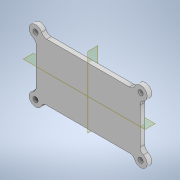
# Autodesk Inventor part: sensor_lid
Saved by Autodesk Inventor 2020 (Build 240168000, 168)
## iProperties
Created: 2020-03-10
Part Number: sensor_lid
Material: Generic
Document SubType Name: Modeling
Designer: Richard
Density: 1 g/cm^3
Appearance: Default
Author: Richard
Autodesk Inventor part; units mm, degrees
ref_plane "YZ Plane" through (0, 0, 0) normal (1, 0, 0) x (0, 1, 0)
ref_plane "XZ Plane" through (0, 0, 0) normal (0, 1, 0) x (-1, 0, 0)
ref_plane "XY Plane" through (0, 0, 0) normal (0, 0, 1) x (1, 0, 0)
sketch "Sketch1" plane through (0, 0, 0) normal (0, 0, 1) x (1, 0, 0)
  line L0 (-172.0273, 68.4234) -> (-119.9573, 68.4234)
  line L1 (-119.9573, 68.4234) -> (-119.9573, 42.0074)
  line L2 (-119.9573, 42.0074) -> (-172.0273, 42.0074)
  line L3 (-172.0273, 42.0074) -> (-172.0273, 68.4234)
  point P0 (0, 0)
  dimension "d0" = 52.07
  dimension "d1" = 26.416
  constraints: 8 end point, 2 parallel, 1 horizontal, 1 perpendicular
  measures "d0" distance of L1.end L2.end
  measures "d1" distance of L0.end L1.end
extrude "Extrusion1" add sketch "Sketch1" along normal blind 2.54
sketch "Sketch2" plane through (0, 0, 2.54) normal (0, 0, 1) x (1, 0, 0)
  line L0 (-119.9573, 68.4234) -> (-172.0273, 68.4234) projected
  line L1 (-119.9573, 68.4234) -> (-172.0273, 68.4234) projected
  line L2 (-172.0273, 68.4234) -> (-172.0273, 42.0074) projected
  line L3 (-172.0273, 42.0074) -> (-119.9573, 42.0074) projected
  line L4 (-119.9573, 42.0074) -> (-119.9573, 68.4234) projected
  line L5 (-174.5673, 39.4674) -> (-174.5673, 70.9634)
  line L6 (-174.5673, 70.9634) -> (-117.4173, 70.9634)
  line L7 (-117.4173, 70.9634) -> (-117.4173, 39.4674)
  line L8 (-117.4173, 39.4674) -> (-174.5673, 39.4674)
  point P0 (0, 0)
  dimension "d4" = 2.54
  constraints: 8 end point, 3 other
  measures "d4" distance between parallel lines of L2 L5
extrude "Extrusion2" add sketch "Sketch2" along normal blind 2.54 contours L4 L3 L2 L0 | L5 L6 L7 L8
fillet "Fillet1" radius 3.175 4 edges at (-174.5673, 39.4674, 3.81) (-117.4173, 39.4674, 3.81) (-117.4173, 70.9634, 3.81) (-174.5673, 70.9634, 3.81)
sketch "Sketch4" plane through (0, 0, 5.08) normal (0, 0, 1) x (1, 0, 0)
  arc A0 (-171.3923, 70.9634) -> (-174.5673, 67.7884) centre (-171.3923, 67.7884) ccw projected
  line L0 (-174.5673, 67.7884) -> (-174.5673, 42.6424) projected
  arc A1 (-174.5673, 42.6424) -> (-171.3923, 39.4674) centre (-171.3923, 42.6424) ccw projected
  line L1 (-171.3923, 39.4674) -> (-120.5923, 39.4674) projected
  arc A2 (-120.5923, 39.4674) -> (-117.4173, 42.6424) centre (-120.5923, 42.6424) ccw projected
  line L2 (-117.4173, 42.6424) -> (-117.4173, 67.7884) projected
  arc A3 (-117.4173, 67.7884) -> (-120.5923, 70.9634) centre (-120.5923, 67.7884) ccw projected
  line L3 (-120.5923, 70.9634) -> (-171.3923, 70.9634) projected
  arc A4 (-171.3923, 70.9634) -> (-174.5673, 67.7884) centre (-171.3923, 67.7884) ccw projected
  line L4 (-174.5673, 67.7884) -> (-174.5673, 42.6424) projected
  arc A5 (-171.3923, 70.9634) -> (-174.5673, 67.7884) centre (-174.9298, 71.3259) ccw
  circle A6 centre (-174.9298, 71.3259) radius 1.3891
  point P0 (0, 0)
  dimension "d12" = 2.7781
  dimension "d13" = 3.556
  constraints: 2 centre point, 2 point on circle, 1 coincident
  measures "d12" diameter of A6
  measures "d13" radius of A5
extrude "Extrusion3" add sketch "Sketch4" against normal up to surface (2.54 mm away) contours A0 A5
ref_plane "Work Plane1" through (-145.9923, 42.6424, 2.54) normal (-1, 0, 0) x (0, 0, 1)
ref_plane "Work Plane2" through (-171.3923, 55.2154, 2.54) normal (0, -1, 0) x (1, 0, 0)
mirror "Mirror1" about plane through (-145.9923, 42.6424, 2.54) normal (-1, 0, 0) of "Extrusion3"
mirror "Mirror2" about plane through (-171.3923, 55.2154, 2.54) normal (0, -1, 0) of "Extrusion3", "Mirror1"
fillet "Fillet2" radius 3.175 8 edges at (-120.5923, 70.9634, 3.81) (-117.4173, 67.7884, 3.81) (-171.3923, 70.9634, 3.81) (-174.5673, 67.7884, 3.81) (-174.5673, 42.6424, 3.81) (-171.3923, 39.4674, 3.81) (-120.5923, 39.4674, 3.81) (-117.4173, 42.6424, 3.81)
body "Solid1"
